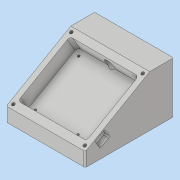
# Autodesk Inventor part: Gehause
Saved by Autodesk Inventor 2018 (Build 220112000, 112)
## iProperties
Created: 2020-10-03
Part Number: Gehause
Material: Generisch
Document SubType Name: Modeling
Designer: marce
Density: 1 g/cm^3
Appearance: Vorgabe
Author: marce
Autodesk Inventor part; units mm, degrees
ref_plane "YZ Plane" through (0, 0, 0) normal (1, 0, 0) x (0, 1, 0)
ref_plane "XZ Plane" through (0, 0, 0) normal (0, 1, 0) x (-1, 0, 0)
ref_plane "XY Plane" through (0, 0, 0) normal (0, 0, 1) x (1, 0, 0)
sketch "Skizze1" plane through (0, 0, 0) normal (0, 0, 1) x (1, 0, 0)
  line L0 (0, 0) -> (85, 0)
  line L1 (85, 0) -> (85, 95)
  line L2 (85, 95) -> (0, 95)
  line L3 (0, 95) -> (0, 0)
  dimension "d0" = 85
  dimension "d1" = 95
  constraints: 8 end point, 2 parallel, 1 horizontal, 1 perpendicular
  measures "d0" distance of L2.end L1.end
  measures "d1" distance of L1.end L0.end
extrude "Extrusion1" add sketch "Skizze1" along normal blind 80
sketch "Skizze2" plane through (85, 0, 0) normal (1, 0, 0) x (0, 0, -1)
  line L0 (0, 0) -> (-80, 0) projected
  line L1 (0, 0) -> (-15, 0)
  line L2 (-15, 0) -> (-55, 69.282)
  line L3 (-55, 69.282) -> (-55, 95)
  line L4 (0, 95) -> (-80, 95) projected
  line L5 (-55, 95) -> (0, 95)
  line L6 (0, 0) -> (0, 95) projected
  line L7 (0, 95) -> (0, 0) projected
  line L8 (0, 95) -> (0, 0)
  dimension "d4" = 15
  dimension "d5" = 80
  dimension "d6" = 120
  constraints: 10 end point, 2 point on line, 1 collinear, 1 perpendicular, 1 vertical
  measures "d4" distance of L0.start L1.end
  measures "d5" distance of L1.end L2.end
  measures "d6" angle of L1 L2
extrude "Extrusion2" cut sketch "Skizze2" against normal through all keep common part
sketch "Skizze3" plane through (0, 0, 15) normal (0, -0.5, 0.866) x (1, 0, 0)
  line L0 (5.5, 72.5) -> (79.5, 72.5)
  line L1 (79.5, 72.5) -> (79.5, 8)
  line L2 (79.5, 8) -> (5.5, 8)
  line L3 (5.5, 8) -> (5.5, 72.5)
  line L4 (85, -7.5) -> (85, 74.7724) projected
  line L5 (85, 80) -> (0, 80) projected
  line L6 (0, 0) -> (85, 0) projected
  point P0 (0, -7.5)
  point P1 (79.5, 40.25)
  point P2 (42.5, 72.5)
  point P3 (42.5, 80)
  dimension "d9" = 74
  dimension "d10" = 64.5
  dimension "d13" = 8
  constraints: 8 end point, 3 midpoint, 2 parallel, 1 horizontal, 1 perpendicular, 1 vertical alignment
  measures "d9" distance of L0.start L0.end
  measures "d10" distance of L0.end L1.end
  measures "d13" distance between parallel lines of L6 L2
extrude "Extrusion3" cut sketch "Skizze3" against normal blind 16.36
sketch "Skizze4" plane through (79.5, 6.9282, 19) normal (-1, 0, 0) x (0, -0.5, 0.866)
  line L0 (-12.26, 3.15) -> (-1.46, 3.15)
  line L1 (-1.46, 3.15) -> (-1.46, 15.35)
  line L2 (-1.46, 15.35) -> (-12.26, 15.35)
  line L3 (-12.26, 15.35) -> (-12.26, 3.15)
  line L4 (-16.36, 64.5) -> (-16.36, 0) projected
  line L5 (0, 0) -> (-16.36, 0) projected
  line L6 (0, 64.5) -> (0, 0) projected
  point P0 (-12.9904, -15.5)
  dimension "d15" = 4.1
  dimension "d16" = 3.15
  dimension "d17" = 12.2
  dimension "d18" = 10.8
  dimension "d19" = 1.46
  constraints: 8 end point, 2 parallel, 1 horizontal, 1 perpendicular
  measures "d15" distance between parallel lines of L4 L3
  measures "d16" distance between parallel lines of L5 L0
  measures "d17" distance of L0.end L1.end
  measures "d18" distance of L1.end L2.end
  measures "d19" distance between parallel lines of L6 L1
extrude "Extrusion4" cut sketch "Skizze4" against normal through all
fillet "Rundung2" radius 1.5 4 edges at (82.25, 26.3517, 16.0575) (82.25, 15.7862, 9.9575) (82.25, 10.3862, 19.3106) (82.25, 20.9517, 25.4106)
sketch "Skizze6" plane through (0, 0, 15) normal (0, -0.5, 0.866) x (1, 0, 0)
  circle A0 centre (4, 4) radius 2.25 projected
  circle A1 centre (4, 76) radius 2.25 projected
  circle A2 centre (81, 76) radius 2.25 projected
  circle A3 centre (81, 4) radius 2.25 projected
  point P0 (0, -7.5)
hole "Bohrung2" at (81, 3.4641, 17) at (81, 65.8179, 53) at (4, 65.8179, 53) at (4, 3.4641, 17) direction (0, 0.5, -0.866) diameter 3.242 depth 11.8 tip angle 118 thread size "M4x0.7" class "6H" standard "ISO Metric profile"
sketch "Skizze7" plane through (0, 95, 0) normal (0, 1, 0) x (1, 0, 0)
  line L0 (85, -55) -> (0, -55) projected
  line L1 (85, 0) -> (85, -55) projected
  line L2 (85, 0) -> (0, 0) projected
  line L3 (0, 0) -> (0, -55) projected
  line L4 (85, 0) -> (85, -55) projected
  line L5 (85, -55) -> (42.5, -55)
  line L6 (42.5, -55) -> (42.5, -41)
  line L7 (42.5, -41) -> (85, -41)
  line L8 (85, -41) -> (85, -55)
  point P0 (0, 0)
  dimension "d37" = 42.5
  dimension "d38" = 14
  constraints: 8 end point, 2 parallel, 1 horizontal, 1 perpendicular
  measures "d37" distance of L6.end L7.end
  measures "d38" distance of L5.end L6.end
hole "Bohrung3" at (42.5, 95, 41) direction (0, -1, 0) diameter 10 end through all
sketch "Skizze8" plane through (0, 8.18, 0.8318) normal (0, -0.5, 0.866) x (1, 0, 0)
  circle A0 centre (11.65, 13) radius 1.6 projected
  circle A1 centre (74.16, 11.255) radius 1.165
  circle A2 centre (73.65, 67) radius 1.6 projected
  circle A3 centre (11.65, 67) radius 1.6 projected
  circle A4 centre (57.65, 13) radius 1.6 projected
  point P0 (0, -7.5)
  constraints: 1 centre point
hole "Bohrung4" at (57.65, 19.4383, 7.3318) at (11.65, 19.4383, 7.3318) at (11.65, 66.2037, 34.3318) at (73.65, 66.2037, 34.3318) direction (0, 0.5, -0.866) diameter 2.459 depth 7 tip angle 118 thread size "M3x0.5" class "6H" standard "ISO Metric profile"
sketch "Skizze9" plane through (0, 95, 0) normal (0, 1, 0) x (1, 0, 0)
  line L0 (72.5, -48) -> (12.5, -48)
  line L1 (12.5, -48) -> (12.5, -7)
  line L2 (12.5, -7) -> (72.5, -7)
  line L3 (72.5, -7) -> (72.5, -48)
  line L4 (85, -55) -> (0, -55) projected
  line L5 (85, 0) -> (0, 0) projected
  point P0 (42.5, -48)
  point P1 (42.5, -55)
  dimension "d54" = 60
  dimension "d55" = 41
  dimension "d56" = 7
  dimension "d57" = 7
  constraints: 8 end point, 2 midpoint, 2 parallel, 1 horizontal, 1 perpendicular, 1 vertical alignment
  measures "d54" distance of L1.end L2.end
  measures "d55" distance of L0.end L1.end
  measures "d56" distance between parallel lines of L4 L0
  measures "d57" distance between parallel lines of L5 L2
hole "Bohrung5" at (12.5, 95, 48) at (12.5, 95, 7) at (72.5, 95, 7) at (72.5, 95, 48) direction (0, -1, 0) diameter 4.917 depth 20 tip angle 118 thread size "M6x1" class "6H" standard "ISO Metric profile"
fillet "Rundung3" radius 1.5 4 edges at (0, 95, 27.5) (0, 0, 7.5) (85, 0, 7.5) (85, 95, 27.5)
fillet "Rundung1" radius 3.1 4 edges at (5.5, 66.8773, 44.165) (79.5, 66.8773, 44.165) (79.5, 11.0187, 11.915) (5.5, 11.0187, 11.915)
